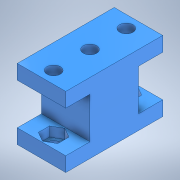
# Autodesk Inventor part: Foot_Spacer
Saved by Autodesk Inventor 2021 (Build 250183000, 183)
## iProperties
Created: 2021-05-18
Part Number: Foot_Spacer
Material: Generic
Document SubType Name: Modeling
Designer: Jorian Brusind
Density: 1 g/cm^3
Appearance: Cyan
Author: Jorian Brusind
Autodesk Inventor part; units mm, degrees
ref_plane "YZ Plane" through (0, 0, 0) normal (1, 0, 0) x (0, 1, 0)
ref_plane "XZ Plane" through (0, 0, 0) normal (0, 1, 0) x (-1, 0, 0)
ref_plane "XY Plane" through (0, 0, 0) normal (0, 0, 1) x (1, 0, 0)
sketch "Sketch6" plane through (0, 0, 0) normal (0, 1, 0) x (-1, 0, 0)
  line L0 (0, 0) -> (20, 0)
  line L1 (20, 0) -> (20, -40)
  line L2 (20, -40) -> (0, -40)
  line L3 (0, -40) -> (0, 0)
  dimension "d39" = 20
  dimension "d40" = 40
  constraints: 8 end point, 2 parallel, 1 horizontal, 1 perpendicular
  measures "d39" distance of L1.end L2.end
  measures "d40" distance of L0.end L1.end
extrude "Extrusion6" add sketch "Sketch6" along normal blind 6
sketch "Sketch8" plane through (0, 0, 0) normal (0, -1, 0) x (1, 0, 0)
  line L0 (0, 0) -> (0, -40) projected
  line L1 (0, -20) -> (-20, -20)
  line L2 (-20, -40) -> (-20, 0) projected
  line L3 (0, -30) -> (-20, -30)
  line L4 (-20, -30) -> (-20, -10)
  line L5 (-20, -10) -> (0, -10)
  line L6 (0, -10) -> (0, -30)
  line L7 (0, -30) -> (-20, -10) construction
  line L8 (-20, -30) -> (0, -10) construction
  point P0 (-10, -20)
  point P1 (0, -10)
  point P2 (-20, -10)
  point P3 (-20, -30)
  point P4 (0, -30)
  dimension "d55" = 20
  dimension "d56" = 20
  constraints: 14 end point, 5 midpoint, 2 parallel, 1 horizontal, 1 perpendicular
  measures "d55" distance of L4.end L5.end
  measures "d56" distance of L3.end L4.end
extrude "Extrusion8" add sketch "Sketch8" along normal blind 17
sketch "Sketch12" plane through (0, -17, 0) normal (0, -1, 0) x (1, 0, 0)
  line L0 (0, -40) -> (-20, -40) projected
  line L1 (0, 0) -> (-20, 0)
  line L2 (-20, 0) -> (-20, -40)
  line L3 (-20, -40) -> (0, -40)
  line L4 (0, -40) -> (0, 0)
  dimension "d78" = 20
  dimension "d79" = 40
  constraints: 8 end point, 2 parallel, 1 horizontal, 1 perpendicular
  measures "d78" distance of L3.end L0.end
  measures "d79" distance of L0.end L1.end
extrude "Extrusion12" add sketch "Sketch12" along normal blind 6
sketch "Sketch7" plane through (0, 6, 0) normal (0, 1, 0) x (1, 0, 0)
  line L0 (-20, 0) -> (0, 0) projected
  line L1 (-10, 0) -> (-10, 20)
  circle A0 centre (-10, 20) radius 2.75
  line L2 (0, 40) -> (-20, 40) projected
  line L3 (-10, 40) -> (-10, 35)
  circle A1 centre (-10, 35) radius 2.75
  line L4 (-20, 40) -> (-20, 0) projected
  line L5 (-20, 20) -> (0, 20)
  line L6 (0, 0) -> (0, 40) projected
  circle A2 centre (-10, 5) radius 2.75
  dimension "d43" = 20
  dimension "d44" = 5.5
  dimension "d45" = 5
  dimension "d46" = 5.5
  dimension "d47" = 5.5
  dimension "d49" = 15
  dimension "d51" = 10
  constraints: 6 end point, 4 midpoint, 3 centre point, 2 coincident, 2 vertical
  measures "d43" distance of L1.start L1.end
  measures "d44" diameter of A0
  measures "d45" distance of L3.start L3.end
  measures "d46" diameter of A1
  measures "d47" diameter of A2
  measures "d49" distance from line of L5 A2.centre
  measures "d51" distance from line of L4 A2.centre
extrude "Extrusion7" cut sketch "Sketch7" against normal through all contours A2 L1 | L1 A2 | L5 L1 A0 | A0 L5 | A0 L1 L5 | A1
sketch "Sketch13" plane through (0, -17, 0) normal (0, 1, 0) x (1, 0, 0)
  circle A0 centre (-10, 5) radius 2.75 projected
  line L0 (-10, 0.3812) -> (-14, 2.6906)
  line L1 (-14, 2.6906) -> (-14, 7.3094)
  line L2 (-14, 7.3094) -> (-10, 9.6188)
  line L3 (-10, 9.6188) -> (-6, 7.3094)
  line L4 (-6, 7.3094) -> (-6, 2.6906)
  line L5 (-6, 2.6906) -> (-10, 0.3812)
  circle A1 centre (-10, 35) radius 2.75 projected
  line L6 (-10, 39.6188) -> (-6, 37.3094)
  line L7 (-6, 37.3094) -> (-6, 32.6906)
  line L8 (-6, 32.6906) -> (-10, 30.3812)
  line L9 (-10, 30.3812) -> (-14, 32.6906)
  line L10 (-14, 32.6906) -> (-14, 37.3094)
  line L11 (-14, 37.3094) -> (-10, 39.6188)
  line L12 (0, 40) -> (0, 30) projected
  point P0 (0, 0)
  dimension "d82" = 8
  dimension "d83" = 8
  constraints: 24 end point, 2 coincident, 1 collinear, 1 parallel, 26 other
  measures "d82" distance between parallel lines of L1 L4
  measures "d83" distance between parallel lines of L10 L7
extrude "Extrusion13" cut sketch "Sketch13" against normal blind 4 contours A0 | L0 L1 L2 L3 L4 L5 | A1 | L6 L7 L8 L9 L10 L11
sketch "Sketch14" plane through (0, -23, 0) normal (0, -1, 0) x (1, 0, 0)
  circle A0 centre (-10, -20) radius 2.75 projected
  line L0 (-5.3812, -20) -> (-7.6906, -24)
  line L1 (-7.6906, -24) -> (-12.3094, -24)
  line L2 (-12.3094, -24) -> (-14.6188, -20)
  line L3 (-14.6188, -20) -> (-12.3094, -16)
  line L4 (-12.3094, -16) -> (-7.6906, -16)
  line L5 (-7.6906, -16) -> (-5.3812, -20)
  line L6 (0, 0) -> (-20, 0) projected
  dimension "d86" = 8
  constraints: 12 end point, 1 coincident, 1 parallel, 13 other
  measures "d86" distance between parallel lines of L1 L4
extrude "Extrusion14" cut sketch "Sketch14" against normal blind 4 contours A0 | L0 L1 L2 L3 L4 L5
body "Solid2"
